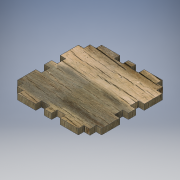
# Autodesk Inventor part: CandleHolder-1
Saved by Autodesk Inventor 2017 (Build 210142000, 142)
## iProperties
Created: 2016-10-20
Part Number: CandleHolder-1
Material: Generic
Document SubType Name: Modeling
Designer: andrew
Density: 1 g/cm^3
Appearance: Driftwood
woodThickness: 0.240 in
glassLength: 3.150 in
glassHeight: 3.180 in
lip: 0.375 in
baseLength: 3.150 in
toothLength: 0.788 in
toothOffset: 0.525 in
lasorTol: 0.003 in
Author: andrew
Autodesk Inventor part; units mm, degrees
ref_plane "YZ Plane" through (0, 0, 0) normal (1, 0, 0) x (0, 1, 0)
ref_plane "XZ Plane" through (0, 0, 0) normal (0, 1, 0) x (-1, 0, 0)
ref_plane "XY Plane" through (0, 0, 0) normal (0, 0, 1) x (1, 0, 0)
sketch "Sketch1" plane through (0, 0, 0) normal (0, 1, 0) x (-1, 0, 0)
  line L0 (40.005, 40.005) -> (-40.005, 40.005)
  line L1 (-40.005, 40.005) -> (-40.005, -40.005)
  line L2 (-40.005, -40.005) -> (-33.3375, -40.005)
  line L3 (40.005, -40.005) -> (40.005, 40.005)
  line L4 (40.005, 40.005) -> (-40.005, -40.005) construction
  line L5 (-40.005, 40.005) -> (40.005, -40.005) construction
  line L6 (46.101, 46.101) -> (-46.101, 46.101)
  line L7 (-46.101, 46.101) -> (-46.101, -46.101)
  line L8 (-46.101, -46.101) -> (-33.3375, -46.101)
  line L9 (46.101, -46.101) -> (46.101, 46.101)
  line L10 (46.101, 46.101) -> (-46.101, -46.101) construction
  line L11 (-46.101, 46.101) -> (46.101, -46.101) construction
  line L12 (33.3375, -40.005) -> (33.3375, -46.101)
  line L13 (13.335, -40.005) -> (13.335, -46.101)
  line L14 (13.335, -40.005) -> (33.3375, -40.005)
  line L15 (33.3375, -46.101) -> (46.101, -46.101)
  line L16 (13.335, -46.101) -> (33.3375, -46.101)
  line L17 (33.3375, -40.005) -> (40.005, -40.005)
  line L18 (-20.9635, 41.5612) -> (22.9239, 41.5612) construction
  line L19 (22.9239, 41.5612) -> (22.9239, 28.3672) construction
  line L20 (22.9239, 28.3672) -> (-20.9635, 28.3672) construction
  line L21 (-20.9635, 28.3672) -> (-20.9635, 41.5612) construction
  line L22 (4.0005, -46.101) -> (4.0005, -40.005)
  line L23 (-4.0005, -46.101) -> (-4.0005, -40.005)
  line L24 (-13.335, -46.101) -> (-13.335, -40.005)
  line L25 (-33.3375, -46.101) -> (-33.3375, -40.005)
  line L26 (4.0005, -40.005) -> (13.335, -40.005)
  line L27 (-4.0005, -40.005) -> (4.0005, -40.005)
  line L28 (-4.0005, -46.101) -> (4.0005, -46.101)
  line L29 (4.0005, -46.101) -> (13.335, -46.101)
  line L30 (-13.335, -46.101) -> (-4.0005, -46.101)
  line L31 (-33.3375, -46.101) -> (-13.335, -46.101)
  line L32 (-33.3375, -40.005) -> (-13.335, -40.005)
  line L33 (-13.335, -40.005) -> (-4.0005, -40.005)
  point P0 (0, 0)
  dimension "baseLength" = 80.01
  dimension "d1" = 80.01
  dimension "d2" = 6.096
  dimension "toothLength" = 20.0025
  dimension "toothOffset" = 13.335
  dimension "d16" = 8.001
  dimension "d17" = 4.0005
  dimension "d18" = 20.0025
  dimension "d19" = 13.335
  constraints: 60 end point, 29 perpendicular, 17 parallel, 4 midpoint, 3 point on line, 2 horizontal, 1 collinear, 2 other
  measures "baseLength" distance of L1.end L3.start
  measures "d1" distance of L0.end L1.end
  measures "d2" distance between parallel lines of L8 L2
  measures "toothLength" distance between parallel lines of L12 L13
  measures "toothOffset" distance from line of L13 point (0, 0)
  measures "d16" distance between parallel lines of L23 L22
  measures "d17" distance from line of point (0, 0) L22
  measures "d18" distance between parallel lines of L25 L24
  measures "d19" distance from line of L24 point (0, 0)
extrude "Extrusion1" add sketch "Sketch1" along normal blind 6.096 contours L3 L17 L14 L26 L27 L33 L32 L2 L1 L0
extrude "Extrusion2" add sketch "Sketch1" along normal blind 6.096 contours L12 L16 L13 L14 | L32 L24 L31 L25 | L22 L28 L23 L27
pattern_circular "Circular Pattern1" count 4 over 360 about axis through (0, -10, 0) along (0, 1, 0) of "Extrusion2"
equation "\"baseLength\" = glassLength"
equation "\"d1\" = baseLength"
equation "\"d2\" = woodThickness"
equation "\"toothLength\" = 0.25 * baseLength"
equation "\"toothOffset\" = 0.666667 * toothLength"
equation "\"d16\" = 0.4 * toothLength"
equation "\"d17\" = 0.5 * d16"
equation "\"d18\" = toothLength"
equation "\"d19\" = toothOffset"
equation "\"d6\" = woodThickness"
equation "\"d8\" = woodThickness"
equation "\"woodThickness\" = 6.096"
equation "\"glassLength\" = 80.01"
equation "\"glassHeight\" = 80.772"
equation "\"lip\" = 9.525"
equation "\"lasorTol\" = 0.0635"
body "Solid1"
